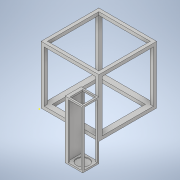
# Autodesk Inventor part: Motor housing 2
Saved by Autodesk Inventor 2021 (Build 250183000, 183)
## iProperties
Created: 2020-10-15
Part Number: Motor housing 2
Material: Generic
Document SubType Name: Modeling
Designer: nabee
Density: 1 g/cm^3
Appearance: Default
Author: nabee
Autodesk Inventor part; units mm, degrees
ref_plane "YZ Plane" through (0, 0, 0) normal (1, 0, 0) x (0, 1, 0)
ref_plane "XZ Plane" through (0, 0, 0) normal (0, 1, 0) x (-1, 0, 0)
ref_plane "XY Plane" through (0, 0, 0) normal (0, 0, 1) x (1, 0, 0)
sketch "Sketch1" plane through (0, 0, 0) normal (0, 0, 1) x (1, 0, 0)
  line L0 (0, 0) -> (380, 0)
  line L1 (380, 0) -> (380, 380)
  line L2 (380, 380) -> (0, 380)
  line L3 (0, 380) -> (0, 0)
  dimension "d0" = 380
  dimension "d1" = 380
  constraints: 8 end point, 2 parallel, 1 horizontal, 1 perpendicular
  measures "d0" distance of L2.end L1.end
  measures "d1" distance of L2.end L0.start
extrude "Extrusion1" add sketch "Sketch1" along normal blind 380
sketch "Sketch2" plane through (0, 0, 380) normal (0, 0, 1) x (1, 0, 0)
  line L0 (30, 350) -> (350, 350)
  line L1 (350, 350) -> (350, 30)
  line L2 (350, 30) -> (30, 30)
  line L3 (30, 30) -> (30, 350)
  line L4 (380, 380) -> (0, 380) projected
  line L5 (0, 380) -> (0, 0) projected
  line L6 (0, 0) -> (380, 0) projected
  line L7 (380, 0) -> (380, 380) projected
  dimension "d4" = 30
  dimension "d5" = 30
  dimension "d6" = 30
  dimension "d7" = 30
  constraints: 8 end point, 2 parallel, 1 horizontal, 1 perpendicular
  measures "d4" distance between parallel lines of L4 L0
  measures "d5" distance between parallel lines of L5 L3
  measures "d6" distance between parallel lines of L6 L2
  measures "d7" distance between parallel lines of L7 L1
extrude "Extrusion2" cut sketch "Sketch2" against normal blind 600 contours L0 L1 L2 L3
sketch "Sketch3" plane through (380, 0, 0) normal (1, 0, 0) x (0, 0, -1)
  line L0 (-350, 350) -> (-30, 350)
  line L1 (-30, 350) -> (-30, 30)
  line L2 (-30, 30) -> (-350, 30)
  line L3 (-350, 30) -> (-350, 350)
  line L4 (0, 380) -> (-380, 380) projected
  line L5 (-380, 0) -> (-380, 380) projected
  line L6 (0, 0) -> (0, 380) projected
  line L7 (0, 0) -> (-380, 0) projected
  dimension "d10" = 30
  dimension "d11" = 30
  dimension "d12" = 30
  dimension "d13" = 30
  constraints: 8 end point, 2 parallel, 1 horizontal, 1 perpendicular
  measures "d10" distance between parallel lines of L4 L0
  measures "d11" distance between parallel lines of L5 L3
  measures "d12" distance between parallel lines of L6 L1
  measures "d13" distance between parallel lines of L7 L2
extrude "Extrusion3" cut sketch "Sketch3" against normal blind 600 contours L0 L1 L2 L3
sketch "Sketch4" plane through (0, 380, 0) normal (0, 1, 0) x (1, 0, 0)
  line L0 (30, -30) -> (30, 0) projected
  line L1 (350, -380) -> (350, -350) projected
  line L2 (30, -30) -> (350, -30)
  line L3 (350, -30) -> (350, -350)
  line L4 (350, -350) -> (30, -350)
  line L5 (30, -350) -> (30, -30)
  point P0 (0, 0)
  constraints: 8 end point, 2 parallel, 1 horizontal, 1 perpendicular
extrude "Extrusion4" cut sketch "Sketch4" against normal blind 600
sketch "Sketch5" plane through (30, 0, 30) normal (1, 0, 0) x (0, 0, -1)
  line L0 (-350, 30) -> (-320, 30) projected
  line L1 (0, 30) -> (0, 0) projected
  line L2 (-320, 30) -> (0, 30)
  line L3 (0, 30) -> (0, 0)
  line L4 (0, 0) -> (-320, 0)
  line L5 (-320, 0) -> (-320, 30)
  point P0 (30, 0)
  constraints: 8 end point, 2 parallel, 1 horizontal, 1 perpendicular
extrude "Extrusion5" add sketch "Sketch5" along normal blind 15
sketch "Sketch6" plane through (350, 0, 30) normal (0, 0, 1) x (1, 0, 0)
  line L0 (-320, 30) -> (-350, 30) projected
  line L1 (0, 30) -> (0, 0) projected
  line L2 (-320, 30) -> (0, 30)
  line L3 (0, 30) -> (0, 0)
  line L4 (0, 0) -> (-320, 0)
  line L5 (-320, 0) -> (-320, 30)
  point P0 (-350, 0)
  constraints: 8 end point, 2 parallel, 1 horizontal, 1 perpendicular
extrude "Extrusion6" add sketch "Sketch6" along normal blind 15
sketch "Sketch7" plane through (350, 0, 350) normal (-1, 0, 0) x (0, 0, 1)
  line L0 (0, 30) -> (-320, 30) projected
  line L1 (0, 0) -> (-305, 0) projected
  line L2 (-320, 30) -> (0, 30)
  line L3 (0, 30) -> (0, 0)
  line L4 (0, 0) -> (-320, 0)
  line L5 (-320, 0) -> (-320, 30)
  point P0 (-350, 0)
  constraints: 8 end point, 2 parallel, 1 horizontal, 1 perpendicular
extrude "Extrusion7" add sketch "Sketch7" along normal blind 15
sketch "Sketch8" plane through (45, 0, 350) normal (0, 0, -1) x (-1, 0, 0)
  line L0 (45, 0) -> (-335, 0) projected
  line L1 (-305, 30) -> (15, 30)
  line L2 (15, 30) -> (15, 0)
  line L3 (15, 0) -> (-305, 0)
  line L4 (-305, 0) -> (-305, 30)
  dimension "d24" = 320
  constraints: 8 end point, 2 parallel, 1 horizontal, 1 perpendicular, 1 point on line
  measures "d24" distance of L2.end L3.end
extrude "Extrusion8" add sketch "Sketch8" along normal blind 15
sketch "Sketch9" plane through (0, 380, 0) normal (0, 1, 0) x (1, 0, 0)
  line L0 (0, -380) -> (380, -380) projected
  line L1 (0, 0) -> (20, 0)
  line L2 (10, -380) -> (0, -380)
  line L3 (0, -380) -> (0, 0)
  line L4 (20, 0) -> (380, 0)
  line L5 (380, 0) -> (380, -10)
  line L6 (380, -10) -> (10, -10)
  line L7 (10, -10) -> (10, -380)
  line L8 (0, -30) -> (0, -350) projected
  dimension "d27" = 10
  dimension "d28" = 10
  constraints: 14 end point, 3 parallel, 2 horizontal, 1 perpendicular, 1 point on line
  measures "d27" distance of L2.start L2.end
  measures "d28" distance of L4.end L5.end
extrude "Extrusion9" cut sketch "Sketch9" against normal blind 900
sketch "Sketch10" plane through (10, 380, 10) normal (0, 1, 0) x (1, 0, 0)
  line L0 (370, 0) -> (360, 0)
  line L1 (360, 0) -> (360, -370)
  line L2 (360, -370) -> (370, -370)
  line L3 (370, -370) -> (370, 0)
  line L4 (0, -370) -> (360, -370)
  line L5 (360, -370) -> (360, -360)
  line L6 (360, -360) -> (0, -360)
  line L7 (0, -360) -> (0, -370)
  point P0 (-10, 10)
  dimension "d31" = 10
  dimension "d32" = 10
  constraints: 16 end point, 4 parallel, 2 horizontal, 2 perpendicular, 1 point on line
  measures "d31" distance of L2.end L1.end
  measures "d32" distance of L6.end L4.start
extrude "Extrusion10" cut sketch "Sketch10" against normal blind 900
sketch "Sketch11" plane through (370, 380, 370) normal (1, 0, 0) x (0, 0, -1)
  line L0 (0, 0) -> (360, 0) projected
  line L1 (0, 0) -> (360, 0)
  line L2 (360, 0) -> (360, -10)
  line L3 (360, -10) -> (0, -10)
  line L4 (0, -10) -> (0, 0)
  line L5 (360, 0) -> (360, -380) projected
  line L6 (0, -380) -> (360, -380)
  line L7 (360, -380) -> (360, -370)
  line L8 (360, -370) -> (0, -370)
  line L9 (0, -370) -> (0, -380)
  point P0 (370, -380)
  dimension "d35" = 10
  dimension "d36" = 10
  constraints: 16 end point, 4 parallel, 2 horizontal, 2 perpendicular, 1 point on line
  measures "d35" distance of L1.end L2.end
  measures "d36" distance of L8.end L6.start
extrude "Extrusion11" cut sketch "Sketch11" against normal blind 900
sketch "Sketch13" plane through (10, 10, 370) normal (0, 0, 1) x (1, 0, 0)
  line L0 (0, 0) -> (360, 0) projected
  line L1 (360, 0) -> (260, 0)
  line L2 (260, 0) -> (260, 500)
  line L3 (260, 500) -> (360, 500)
  line L4 (360, 500) -> (360, 0)
  point P0 (-10, -10)
  point P1 (260, 0)
  dimension "d41" = 100
  dimension "d42" = 500
  constraints: 8 end point, 2 parallel, 1 horizontal, 1 perpendicular
  measures "d41" distance of L2.end L3.end
  measures "d42" distance of L1.end L2.end
extrude "Extrusion13" add sketch "Sketch13" along normal blind 100
sketch "Sketch14" plane through (270, 510, 370) normal (0, 1, 0) x (1, 0, 0)
  line L0 (10, -10) -> (90, -10)
  line L1 (90, -10) -> (90, -90)
  line L2 (90, -90) -> (10, -90)
  line L3 (10, -90) -> (10, -10)
  line L4 (100, 0) -> (0, 0) projected
  line L5 (0, 0) -> (0, -100) projected
  line L6 (100, -100) -> (0, -100) projected
  line L7 (100, 0) -> (100, -100) projected
  point P0 (-270, 370)
  dimension "d45" = 10
  dimension "d46" = 10
  dimension "d47" = 10
  dimension "d48" = 10
  constraints: 8 end point, 2 parallel, 1 horizontal, 1 perpendicular
  measures "d45" distance between parallel lines of L4 L0
  measures "d46" distance between parallel lines of L5 L3
  measures "d47" distance between parallel lines of L6 L2
  measures "d48" distance between parallel lines of L7 L1
extrude "Extrusion14" cut sketch "Sketch14" against normal blind 900 contours L0 L1 L2 L3
sketch "Sketch15" plane through (10, 10, 470) normal (0, 0, 1) x (1, 0, 0)
  line L0 (270, 500) -> (270, 0) projected
  line L1 (360, 20) -> (340, 20) projected
  line L2 (270, 490) -> (350, 490)
  line L3 (350, 490) -> (350, 20)
  line L4 (350, 20) -> (270, 20)
  line L5 (270, 20) -> (270, 490)
  line L6 (360, 500) -> (260, 500) projected
  point P0 (-10, -10)
  point P1 (270, 20)
  dimension "d51" = 10
  constraints: 8 end point, 2 parallel, 1 horizontal, 1 midpoint, 1 perpendicular, 1 point on line
  measures "d51" distance between parallel lines of L6 L2
extrude "Extrusion15" cut sketch "Sketch15" against normal blind 100
sketch "Sketch16" plane through (370, 10, 10) normal (1, 0, 0) x (0, 0, -1)
  line L0 (-450, 490) -> (-370, 490)
  line L1 (-370, 490) -> (-370, 20)
  line L2 (-370, 20) -> (-450, 20)
  line L3 (-450, 20) -> (-450, 490)
  line L4 (-360, 500) -> (-460, 500) projected
  line L5 (-460, 0) -> (-460, 500) projected
  line L6 (-360, 360) -> (-360, 500) projected
  line L7 (0, 0) -> (-460, 0) projected
  point P0 (10, -10)
  dimension "d54" = 10
  dimension "d55" = 10
  dimension "d56" = 10
  dimension "d57" = 20
  constraints: 8 end point, 2 parallel, 1 horizontal, 1 perpendicular
  measures "d54" distance between parallel lines of L4 L0
  measures "d55" distance between parallel lines of L5 L3
  measures "d56" distance between parallel lines of L6 L1
  measures "d57" distance between parallel lines of L7 L2
extrude "Extrusion16" cut sketch "Sketch16" against normal blind 100
sketch "Sketch17" plane through (10, 10, 10) normal (0, -1, 0) x (1, 0, 0)
  line L0 (270, 450) -> (350, 450) projected
  line L1 (270, 370) -> (350, 370) projected
  line L2 (270, 450) -> (350, 450)
  line L3 (350, 450) -> (350, 370)
  line L4 (350, 370) -> (270, 370)
  line L5 (270, 370) -> (270, 450)
  point P0 (-10, -10)
  point P1 (350, 450)
  constraints: 8 end point, 2 parallel, 1 horizontal, 1 perpendicular
extrude "Extrusion17" add sketch "Sketch17" against normal blind 20
sketch "Sketch19" plane through (370, 10, 10) normal (1, 0, 0) x (0, 0, -1)
  line L0 (-360, 500) -> (-460, 500) projected
  line L1 (-360, 490) -> (-360, 360) projected
  line L2 (-460, 500) -> (-360, 500)
  line L3 (-360, 500) -> (-360, 420)
  line L4 (-360, 420) -> (-460, 420)
  line L5 (-460, 420) -> (-460, 500)
  point P0 (10, -10)
  dimension "d65" = 80
  constraints: 8 end point, 2 parallel, 1 horizontal, 1 perpendicular, 1 point on line
  measures "d65" distance of L4.end L0.end
extrude "Extrusion19" cut sketch "Sketch19" against normal blind 8900
sketch "Sketch20" plane through (370, 10, 10) normal (1, 0, 0) x (0, 0, -1)
  line L0 (-460, 420) -> (-450, 420) projected
  line L1 (-360, 360) -> (-360, 20) projected
  line L2 (-460, 420) -> (-360, 420)
  line L3 (-360, 420) -> (-360, 360)
  line L4 (-360, 360) -> (-460, 360)
  line L5 (-460, 360) -> (-460, 420)
  point P0 (10, -10)
  constraints: 8 end point, 2 parallel, 1 horizontal, 1 perpendicular
extrude "Extrusion20" cut sketch "Sketch20" against normal blind 8900
sketch "Sketch21" plane through (270, 370, 380) normal (0, 0, 1) x (1, 0, 0)
  line L0 (10, -20) -> (10, 0) projected
  line L1 (0, 0) -> (10, 0)
  line L2 (10, 0) -> (10, -20)
  line L3 (10, -20) -> (0, -20)
  line L4 (0, -20) -> (0, 0)
  point P0 (-270, -370)
  constraints: 8 end point, 2 parallel, 1 horizontal, 1 perpendicular
extrude "Extrusion21" add sketch "Sketch21" along normal up to surface (80 mm away)
sketch "Sketch22" plane through (280, 30, 470) normal (1, 0, 0) x (0, 0, -1)
  line L0 (0, 340) -> (10, 340)
  line L1 (10, 340) -> (10, 320)
  line L2 (10, 320) -> (0, 320)
  line L3 (0, 320) -> (0, 340)
  point P0 (470, -30)
  dimension "d72" = 20
  constraints: 8 end point, 2 parallel, 1 horizontal, 1 perpendicular
  measures "d72" distance of L0.end L1.end
extrude "Extrusion22" add sketch "Sketch22" along normal up to surface (80 mm away)
sketch "Sketch23" plane through (370, 10, 10) normal (1, 0, 0) x (0, 0, -1)
  line L0 (-370, 20) -> (-370, 360) projected
  line L1 (-450, 360) -> (-370, 360)
  line L2 (-370, 360) -> (-370, 340)
  line L3 (-370, 340) -> (-450, 340)
  line L4 (-450, 340) -> (-450, 360)
  point P0 (10, -10)
  dimension "d75" = 20
  constraints: 8 end point, 2 parallel, 1 horizontal, 1 perpendicular, 1 point on line
  measures "d75" distance of L3.end L1.start
extrude "Extrusion23" add sketch "Sketch23" against normal blind 10
sketch "Sketch26" plane through (10, 10, 10) normal (0, -1, 0) x (1, 0, 0)
  line L0 (260, 460) -> (360, 460) projected
  line L1 (360, 0) -> (360, 460) projected
  line L2 (260, 460) -> (360, 460)
  line L3 (360, 460) -> (360, 360)
  line L4 (360, 360) -> (260, 360)
  line L5 (260, 360) -> (260, 460)
  point P0 (-10, -10)
  dimension "d86" = 100
  constraints: 8 end point, 2 parallel, 1 horizontal, 1 perpendicular, 1 point on line
  measures "d86" distance of L4.end L0.start
extrude "Extrusion26" add sketch "Sketch26" along normal blind 120
sketch "Sketch30" plane through (10, 10, 470) normal (0, 0, 1) x (1, 0, 0)
  line L0 (360, 360) -> (260, 360) projected
  line L1 (260, 340) -> (260, 20) projected
  line L2 (360, 360) -> (260, 360)
  line L3 (260, 360) -> (260, 240)
  line L4 (260, 240) -> (360, 240)
  line L5 (360, 240) -> (360, 360)
  point P0 (-10, -10)
  dimension "d96" = 120
  constraints: 8 end point, 2 parallel, 1 horizontal, 1 perpendicular, 1 point on line
  measures "d96" distance of L4.end L0.start
extrude "Extrusion30" cut sketch "Sketch30" against normal up to surface (100 mm away)
sketch "Sketch31" plane through (370, 10, 10) normal (1, 0, 0) x (0, 0, -1)
  line L0 (-450, 240) -> (-450, 20) projected
  line L1 (-450, 20) -> (-370, 20)
  line L2 (-370, 20) -> (-370, -110)
  line L3 (-370, -110) -> (-450, -110)
  line L4 (-450, -110) -> (-450, 20)
  line L5 (-360, -120) -> (-460, -120) projected
  point P0 (10, -10)
  dimension "d99" = 10
  constraints: 8 end point, 2 parallel, 1 horizontal, 1 perpendicular
  measures "d99" distance between parallel lines of L5 L3
extrude "Extrusion31" cut sketch "Sketch31" against normal blind 200
sketch "Sketch32" plane through (10, 10, 470) normal (0, 0, 1) x (1, 0, 0)
  line L0 (350, 20) -> (270, 20) projected
  line L1 (270, 20) -> (350.1391, 20)
  line L2 (350.1391, 20) -> (350.1391, -110)
  line L3 (350.1391, -110) -> (270, -110)
  line L4 (270, -110) -> (270, 20)
  line L5 (360, -120) -> (260, -120) projected
  point P0 (-10, -10)
  point P1 (350, 20)
  dimension "d102" = 10
  constraints: 8 end point, 2 parallel, 1 horizontal, 1 perpendicular
  measures "d102" distance between parallel lines of L5 L3
extrude "Extrusion32" cut sketch "Sketch32" against normal blind 100
sketch "Sketch33" plane through (270, 250, 380) normal (0, 0, 1) x (1, 0, 0)
  line L0 (0, 0) -> (10, 0) projected
  line L1 (10, -350) -> (10, 0) projected
  line L2 (0, 0) -> (10, 0)
  line L3 (10, 0) -> (10, -10)
  line L4 (10, -10) -> (0, -10)
  line L5 (0, -10) -> (0, 0)
  point P0 (-270, -250)
  dimension "d105" = 10
  constraints: 8 end point, 2 parallel, 1 horizontal, 1 perpendicular, 1 point on line
  measures "d105" distance of L4.end L0.start
extrude "Extrusion33" add sketch "Sketch33" along normal up to surface (80 mm away)
sketch "Sketch34" plane through (280, 10, 370) normal (1, 0, 0) x (0, 0, -1)
  line L0 (-90, 240) -> (-90, 20) projected
  line L1 (-100, 240) -> (-90, 240)
  line L2 (-90, 240) -> (-90, 230)
  line L3 (-90, 230) -> (-100, 230)
  line L4 (-100, 230) -> (-100, 240)
  line L5 (0, 240) -> (-100, 240) projected
  line L6 (-10, 20) -> (-10, 240) projected
  line L7 (0, 240) -> (-10, 240)
  line L8 (-10, 240) -> (-10, 230)
  line L9 (-10, 230) -> (0, 230)
  line L10 (0, 230) -> (0, 240)
  point P0 (370, -10)
  point P1 (-90, 240)
  dimension "d108" = 10
  constraints: 16 end point, 4 parallel, 2 horizontal, 2 perpendicular, 2 point on line
  measures "d108" distance of L3.end L1.start
extrude "Extrusion34" add sketch "Sketch34" along normal up to surface (90 mm away)
sketch "Sketch35" plane through (280, 250, 380) normal (0, 0, 1) x (1, 0, 0)
  line L0 (0, 0) -> (90, 0) projected
  line L1 (80, -10) -> (80, -220) projected
  line L2 (90, 0) -> (80, 0)
  line L3 (80, 0) -> (80, -10)
  line L4 (80, -10) -> (90, -10)
  line L5 (90, -10) -> (90, 0)
  point P0 (-280, -250)
  constraints: 8 end point, 2 parallel, 1 horizontal, 1 perpendicular
extrude "Extrusion35" add sketch "Sketch35" along normal up to surface (80 mm away)
sketch "Sketch36" plane through (370, -100, 460) normal (0, 1, 0) x (1, 0, 0)
  line L0 (-340, 90) -> (-100, 90) projected
  line L1 (0, -10) -> (-100, -10) projected
  line L2 (-100, 90) -> (0, -10)
  circle A0 centre (-50, 40) radius 39
  point P0 (-370, 460)
  dimension "d113" = 78
  constraints: 2 end point, 1 centre point, 1 midpoint
  measures "d113" diameter of A0
extrude "Extrusion36" cut sketch "Sketch36" against normal blind 5
sketch "Sketch41" plane through (30, 350, 370) normal (0, 0, 1) x (1, 0, 0)
  point P0 (-30, -350)
sketch "Sketch42" plane through (270, 250, 470) normal (0, 1, 0) x (1, 0, 0)
  line L0 (-240, 100) -> (0, 100) projected
  line L1 (0, 100) -> (-10, 100)
  line L2 (-10, 100) -> (-10, 0)
  line L3 (-10, 0) -> (0, 0)
  line L4 (0, 0) -> (0, 100)
  point P0 (-270, 470)
  dimension "d119" = 10
  constraints: 8 end point, 2 parallel, 1 horizontal, 1 perpendicular
  measures "d119" distance of L3.end L2.end
extrude "Extrusion37" add sketch "Sketch42" against normal up to surface (360 mm away)
body "Solid1"
